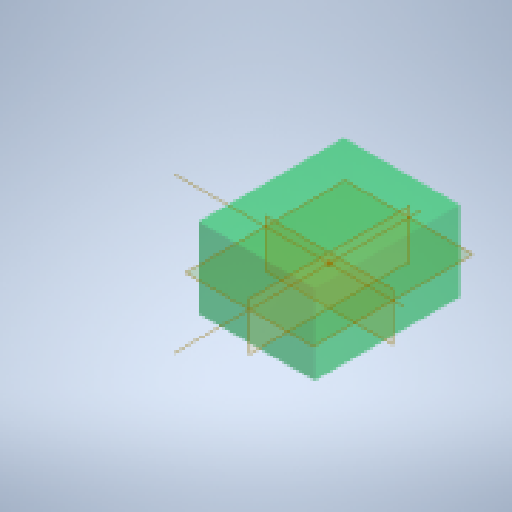
# Autodesk Inventor part: KTN1
Saved by Autodesk Inventor 2026 (Build 300175050, 175E)
## iProperties
Created: 2024-08-20
Part Number: KTN1
Material: Generic
Document SubType Name: Modeling
Designer: User
Density: 1 g/cm^3
Appearance: Default
Author: User
Autodesk Inventor part; units mm, degrees
ref_plane "YZ Plane" through (0, 0, 0) normal (1, 0, 0) x (0, 1, 0)
ref_plane "XZ Plane" through (0, 0, 0) normal (0, 1, 0) x (-1, 0, 0)
ref_plane "XY Plane" through (0, 0, 0) normal (0, 0, 1) x (1, 0, 0)
sketch "Sketch1" plane through (0, 0, 0) normal (0, 1, 0) x (-1, 0, 0)
  line L0 (4, -5) -> (-4, -5)
  line L1 (-4, -5) -> (-4, 5)
  line L2 (-4, 5) -> (4, 5)
  line L3 (4, 5) -> (4, -5)
  line L4 (4, -5) -> (-4, 5) construction
  line L5 (-4, -5) -> (4, 5) construction
  point P0 (0, 0)
  dimension "d0" = 8
  dimension "d1" = 10
  constraints: 12 end point, 2 midpoint, 2 parallel, 1 horizontal, 1 perpendicular
  measures "d0" distance of L1.end L2.end
  measures "d1" distance of L0.end L1.end
extrude "Extrusion1" add sketch "Sketch1" along normal blind 5.5
ref_plane "Work Plane2" through (-4, 0, 0) normal (0, 0, 1) x (1, 0, 0)
ref_plane "Work Plane1" through (0, 2.5, 0) normal (0, -1, 0) x (1, 0, 0)
ref_plane "Work Plane3" through (0, 0, 5) normal (1, 0, 0) x (0, 0, -1)
body "Solid1"
